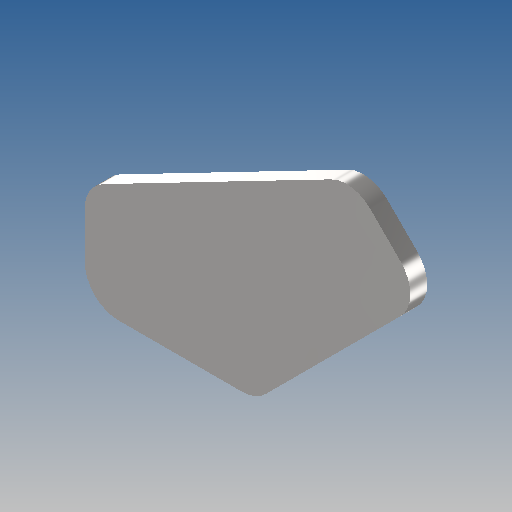
# Autodesk Inventor part: PWTR-0089
Saved by Autodesk Inventor 2021.1 (Build 251245000, 245)
## iProperties
Created: 2020-08-28
Part Number: PWTR-0089
Material: Stainless Steel
Document SubType Name: Sheet Metal
Designer: alid
Density: 8 g/cm^3
Sheet Metal Rule: Default_mm
Appearance: Semi-Polished
Flat Pattern Width: 5.58038 cm
Flat Pattern Length: 10.2678 cm
Flat Pattern Area: 57.2981 cm^2
Sheet Metal Width: 55.804 mm
Sheet Metal Length: 102.678 mm
Sheet Metal Area: 5729.806 mm^2
Description: Arm Bracket Brace
Author: alid
Revision Number: A
Autodesk Inventor part; units mm, degrees
ref_plane "YZ Plane" through (0, 0, 0) normal (1, 0, 0) x (0, 1, 0)
ref_plane "XZ Plane" through (0, 0, 0) normal (0, 1, 0) x (-1, 0, 0)
ref_plane "XY Plane" through (0, 0, 0) normal (0, 0, 1) x (1, 0, 0)
sketch "Sketch1" plane through (0, 0, 0) normal (0, 1, 0) x (-1, 0, 0)
  line L0 (0, 25) -> (0, -25)
  line L1 (0, 25) -> (-59.2893, 25) construction
  line L2 (-59.2893, 25) -> (-143.6396, 109.3503) construction
  line L3 (-143.6396, 109.3503) -> (-178.9949, 73.9949)
  line L4 (-178.9949, 73.9949) -> (-80, -25)
  line L5 (-80, -25) -> (0, -25)
  line L6 (-25, 25) -> (-25, -25)
  line L7 (-97.6777, 63.3883) -> (-133.033, 28.033)
  line L8 (-25, 15) -> (-104.7487, 56.3173)
  line L9 (-25, -15) -> (-75.8579, -15)
  line L10 (-75.8579, -15) -> (-125.9619, 35.1041)
  point P0 (0, 0)
  point P1 (0, 0)
  dimension "d0" = 50
  dimension "d1" = 80
  dimension "d2" = 135
  dimension "d3" = 140
  dimension "d4" = 50
  dimension "d37" = 25
  dimension "d38" = 65
  dimension "d39" = 10
  dimension "d40" = 10
  dimension "d41" = 10
  dimension "d42" = 10
  measures "d0" distance of L0.start L0.end
  measures "d1" distance of L4.end L0.end
  measures "d2" angle of L4 L5
  measures "d3" distance of L3.end L4.end
  measures "d4" distance between parallel lines of L4 L2
  measures "d37" distance from line of L6.start L0
  measures "d38" distance between parallel lines of L3 L7
  measures "d39" distance between parallel lines of L5 L9
  measures "d40" distance between parallel lines of L4 L10
  measures "d41" distance from line of L8.start L1
  measures "d42" distance of L7.start L8.end
extrude "Plate1" add sketch "Sketch1" along normal blind 5 contours L7 L8 L6 L9 L10
fillet "Corner Round1" radius 10 5 edges at (25, 2.5, -15) (25, 2.5, 15) (104.7487, 2.5, 56.3173) (125.9619, 2.5, 35.1041) (75.8579, 2.5, -15)
equation "\"d4\" = d0"
equation "\"d40\" = d39"
equation "\"d41\" = d39"
equation "\"d42\" = d41"
equation "\"d5\" = Thickness"
equation "\"BendRadius\" = Thickness"
equation "\"BendReliefWidth\" = Thickness"
equation "\"BendReliefDepth\" = 0.5 * Thickness"
equation "\"TransitionRadius\" = BendRadius"
equation "\"JacobiRadiusSize\" = BendRadius"
equation "\"GapSize\" = Thickness"
equation "\"Thickness\" = 5"
body "Solid1"
